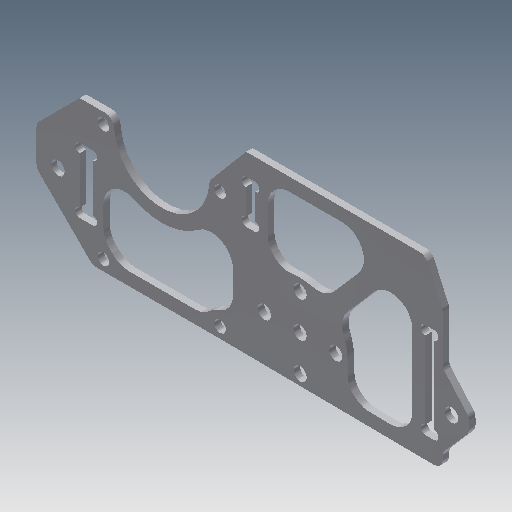
# Autodesk Inventor part: 付け根_メインフレーム_1_1
Saved by Autodesk Inventor 2017.3 (Build 213256000, 256)
## iProperties
Created: 2016-04-30
Part Number: 付け根_メインフレーム_1_1
Material: アルミニウム 2014-T4
Document SubType Name: Modeling
Designer: hiroaki
Density: 2.8 g/cm^3
Appearance: サテン
Mass: 7.66121 g
Surface Area: 47.3307 cm^2
Volume: 2.73615 cm^3
d0: 1.000 ul
d1: 3.000 mm
d2: 15.000 mm
d3: 5.000 mm
d4: 0.025 mm
d5: 2.100 mm
d6: 3.100 mm
d8: 15.000 mm
d9: 11.000 mm
d10: 2.000 mm
d11: 10.000 mm
d12: 5.000 mm
d13: 6.100 mm
d14: 1.000 mm
d15: 0.025 mm
d16: 2.100 mm
d17: 22.000 mm
d18: 5.000 mm
d19: 5.000 mm
d20: 15.000 mm
d21: 1.000 mm
d22: 27.000 mm
d23: 4.000 mm
d24: 2.000 mm
d25: 8.500 mm
d26: 8.500 mm
d28: 0.025 mm
d29: 2.100 mm
d30: 3.100 mm
d31: 1.500 mm
d32: 0.00 deg
d33: 2.100 mm
d34: 6.000 ul
d36: 360.00 deg
d38: 5.600 mm
d39: 0.250 mm
d40: 0.00 deg
Author: hiroaki
Autodesk Inventor part; units mm, degrees
ref_plane "YZ Plane" through (0, 0, 0) normal (1, 0, 0) x (0, 1, 0)
ref_plane "XZ Plane" through (0, 0, 0) normal (0, 1, 0) x (-1, 0, 0)
ref_plane "XY Plane" through (0, 0, 0) normal (0, 0, 1) x (1, 0, 0)
derived "下半身全体像_1_1.ipt"
sketch "スケッチ1" plane through (0, 0, 0) normal (0, 0, 1) x (1, 0, 0)
  circle A0 centre (0, 0) radius 10.5 construction
  line L0 (0, 0) -> (-12, 0) construction
  arc A1 (0, 16) -> (-12, 10.583) centre (0, 0) ccw construction
  arc A2 (-12, -10.583) -> (0, -16) centre (0, 0) ccw construction
  line L1 (0, 16) -> (39.5, 16) construction
  line L2 (39.5, 16) -> (39.5, -16) construction
  line L3 (39.5, -16) -> (0, -16) construction
  circle A3 centre (1, 13.5) radius 1.35 projected
  circle A4 centre (1, -13.5) radius 1.35 projected
  circle A5 centre (28, 13.5) radius 1.35 projected
  circle A6 centre (28, -13.5) radius 1.35 projected
  line L4 (1, 13.5) -> (1, -13.5) construction
  line L5 (1, -13.5) -> (28, -13.5) construction
  line L6 (1, 13.5) -> (28, 13.5) construction
  line L7 (28, 13.5) -> (28, -13.5) construction
  line L8 (0, 0) -> (1, 0) construction
  line L9 (32, 120) -> (32, 20) construction
  line L10 (0, 0) -> (0, 0) construction
  circle A7 centre (32, 120) radius 4.05 construction
  line L11 (0, 140) -> (0, 40) construction
  circle A8 centre (0, 40) radius 4.05 projected
  line L12 (0, 0) -> (0, -100) construction
  line L13 (32, 20) -> (32, -80) construction
  line L14 (0, 0) -> (0, 40) construction
  circle A9 centre (32, 20) radius 6.5 construction
  line L15 (32, 23.5218) -> (35.05, 21.7609) construction
  line L16 (35.05, 21.7609) -> (35.05, 18.2391) construction
  line L17 (35.05, 18.2391) -> (32, 16.4782) construction
  line L18 (32, 16.4782) -> (28.95, 18.2391) construction
  line L19 (28.95, 18.2391) -> (28.95, 21.7609) construction
  line L20 (28.95, 21.7609) -> (32, 23.5218) construction
  line L21 (21.5, 152) -> (61, 152) construction
  line L22 (61, 152) -> (61, 100.5) construction
  line L23 (61, 100.5) -> (21.5, 100.5) construction
  line L24 (21.5, 100.5) -> (21.5, 152) construction
  line L25 (21.5, 140) -> (61, 140) construction
  line L26 (16, 150.5) -> (66.5, 150.5) construction
  line L27 (66.5, 150.5) -> (66.5, 129.5) construction
  line L28 (66.5, 129.5) -> (16, 129.5) construction
  line L29 (16, 129.5) -> (16, 150.5) construction
  circle A10 centre (0, 140) radius 10.5 construction
  line L30 (-13.5, 139) -> (13.5, 139) construction
  line L31 (13.5, 139) -> (13.5, 112) construction
  line L32 (13.5, 112) -> (-13.5, 112) construction
  line L33 (-13.5, 112) -> (-13.5, 139) construction
  circle A11 centre (-13.5, 139) radius 1.35 projected
  circle A12 centre (13.5, 139) radius 1.35 projected
  circle A13 centre (-13.5, 112) radius 1.35 projected
  circle A14 centre (13.5, 112) radius 1.35 projected
  line L34 (-12, 10.583) -> (-12, -10.583) construction
  circle A15 centre (0, -100) radius 4.05 projected
  circle A16 centre (32, -80) radius 4.05 projected
  circle A17 centre (0, -100) radius 10.5 construction
  line L35 (32, -80) -> (0, -100) construction
  line L36 (45, -60.5) -> (77.5, -60.5) construction
  line L37 (77.5, -60.5) -> (77.5, -112) construction
  line L38 (77.5, -112) -> (45, -112) construction
  line L39 (45, -112) -> (45, -60.5) construction
  line L40 (45, -100) -> (77.5, -100) construction
  line L41 (39.5, -89.5) -> (83, -89.5) construction
  line L42 (83, -89.5) -> (83, -110.5) construction
  line L43 (83, -110.5) -> (39.5, -110.5) construction
  line L44 (39.5, -110.5) -> (39.5, -89.5) construction
  line L45 (1, -86.5) -> (28, -86.5) construction
  line L46 (28, -86.5) -> (28, -113.5) construction
  line L47 (28, -113.5) -> (1, -113.5) construction
  line L48 (1, -113.5) -> (1, -86.5) construction
  circle A18 centre (1, -86.5) radius 1.35 projected
  circle A19 centre (1, -113.5) radius 1.35 projected
  circle A20 centre (28, -113.5) radius 1.35 projected
  circle A21 centre (28, -86.5) radius 1.35 projected
  circle A22 centre (32, 20) radius 4.05 projected
  circle A23 centre (32, 20) radius 4.05 projected
  line L49 (10.583, 152) -> (-10.583, 152) construction
  line L50 (16, 140) -> (16, 100.5) construction
  line L51 (16, 100.5) -> (-16, 100.5) construction
  line L52 (-16, 100.5) -> (-16, 140) construction
  arc A24 (16, 140) -> (10.583, 152) centre (0, 140) ccw construction
  arc A25 (-10.583, 152) -> (-16, 140) centre (0, 140) ccw construction
  line L53 (-12, -89.417) -> (-12, -110.583) construction
  line L54 (0, -84) -> (39.5, -84) construction
  line L55 (39.5, -84) -> (39.5, -116) construction
  line L56 (39.5, -116) -> (0, -116) construction
  arc A26 (0, -84) -> (-12, -89.417) centre (0, -100) ccw construction
  arc A27 (-12, -110.583) -> (0, -116) centre (0, -100) ccw construction
  circle A28 centre (-8.5, 0) radius 1.35 projected
  circle A29 centre (0, 0) radius 8.5 construction
  line L57 (35.05, 121.7609) -> (35.05, 118.2391) construction
  line L58 (35.05, 118.2391) -> (32, 116.4782) construction
  line L59 (32, 116.4782) -> (28.95, 118.2391) construction
  line L60 (28.95, 118.2391) -> (28.95, 121.7609) construction
  line L61 (28.95, 121.7609) -> (32, 123.5218) construction
  line L62 (32, 123.5218) -> (35.05, 121.7609) construction
  line L63 (0, 152) -> (0, 140) construction
  line L64 (0, 140) -> (0, 139) construction
  line L65 (-19, 132.5) -> (-16, 132.5) construction
  line L66 (-16, 132.5) -> (-16, 117.5) construction
  line L67 (-16, 117.5) -> (-19, 117.5) construction
  line L68 (-19, 117.5) -> (-19, 132.5) construction
  line L69 (-19, 137.5) -> (-16, 137.5) construction
  line L70 (-16, 137.5) -> (-16, 112.5) construction
  line L71 (-16, 112.5) -> (-19, 112.5) construction
  line L72 (-19, 112.5) -> (-19, 137.5) construction
  line L73 (-15.975, 132.525) -> (-19.025, 132.525) construction
  line L74 (-19.025, 132.525) -> (-19.025, 117.475) construction
  line L75 (-19.025, 117.475) -> (-15.975, 117.475) construction
  line L76 (-15.975, 117.475) -> (-15.975, 132.525) construction
  circle A30 centre (-19.025, 131.475) radius 1.05 construction
  arc A31 (-19.025, 132.525) -> (-19.025, 130.425) centre (-19.025, 131.475) ccw
  line L77 (-19.025, 132.525) -> (-15.975, 132.525)
  arc A32 (-15.975, 130.425) -> (-15.975, 132.525) centre (-15.975, 131.475) ccw
  line L78 (-17.5, 132.525) -> (-17.5, 117.475) construction
  line L79 (-19, 125) -> (-16, 125) construction
  line L80 (-19.025, 130.425) -> (-19.025, 119.575)
  line L81 (-15.975, 130.425) -> (-15.975, 119.575)
  arc A33 (-19.025, 119.575) -> (-19.025, 117.475) centre (-19.025, 118.525) ccw
  arc A34 (-15.975, 117.475) -> (-15.975, 119.575) centre (-15.975, 118.525) ccw
  line L82 (-15.975, 117.475) -> (-19.025, 117.475)
  circle A35 centre (32, 120) radius 1.55
  circle A36 centre (-13.5, 139) radius 2.5 construction
  arc A37 (-10.8799, 138.3793) -> (10.8799, 138.3793) centre (0, 140) ccw
  line L83 (61, 136) -> (63, 136) construction
  line L84 (63, 136) -> (63, 114) construction
  line L85 (63, 114) -> (61, 114) construction
  line L86 (61, 114) -> (61, 136) construction
  line L87 (19.5, 145) -> (21.5, 145) construction
  line L88 (21.5, 145) -> (21.5, 135) construction
  line L89 (21.5, 135) -> (19.5, 135) construction
  line L90 (19.5, 135) -> (19.5, 145) construction
  line L91 (19.5, 150) -> (21.5, 150) construction
  line L92 (21.5, 150) -> (21.5, 130) construction
  line L93 (21.5, 130) -> (19.5, 130) construction
  line L94 (19.5, 130) -> (19.5, 150) construction
  line L95 (10.8799, 138.3793) -> (11.1317, 140.0691)
  circle A38 centre (13.5, 139) radius 2.5 construction
  line L96 (19.5, 150) -> (61, 150)
  line L97 (67.05, 124.5218) -> (70.1, 122.7609) construction
  line L98 (70.1, 122.7609) -> (70.1, 119.2391) construction
  line L99 (70.1, 119.2391) -> (67.05, 117.4782) construction
  line L100 (67.05, 117.4782) -> (64, 119.2391) construction
  line L101 (64, 119.2391) -> (64, 122.7609) construction
  line L102 (64, 122.7609) -> (67.05, 124.5218) construction
  line L103 (21.525, 145.025) -> (19.475, 145.025) construction
  line L104 (19.475, 145.025) -> (19.475, 134.975) construction
  line L105 (19.475, 134.975) -> (21.525, 134.975) construction
  line L106 (21.525, 134.975) -> (21.525, 145.025) construction
  circle A39 centre (19.475, 143.975) radius 1.05 construction
  arc A40 (19.475, 145.025) -> (19.475, 142.925) centre (19.475, 143.975) ccw
  line L107 (20.5, 134.975) -> (20.5, 145.025) construction
  line L108 (19.5, 140) -> (21.5, 140) construction
  line L109 (19.475, 145.025) -> (21.525, 145.025)
  arc A41 (21.525, 142.925) -> (21.525, 145.025) centre (21.525, 143.975) ccw
  line L110 (21.525, 142.925) -> (21.525, 137.075)
  line L111 (19.475, 142.925) -> (19.475, 137.075)
  arc A42 (19.475, 137.075) -> (19.475, 134.975) centre (19.475, 136.025) ccw
  line L112 (19.475, 134.975) -> (21.525, 134.975)
  arc A43 (21.525, 134.975) -> (21.525, 137.075) centre (21.525, 136.025) ccw
  line L113 (61, 150) -> (65, 141)
  line L114 (65, 141) -> (65, 129.5)
  line L115 (65, 141) -> (61, 141) construction
  line L116 (65, 129.5) -> (71.1, 122.5204)
  line L117 (71.1, 122.5204) -> (71.1, 119.4796)
  line L118 (71.1, 119.4796) -> (65, 112.5)
  circle A44 centre (67.05, 121) radius 4.05 construction
  line L119 (61, 109) -> (64.2641, 109) construction
  line L120 (63, 125) -> (61, 125) construction
  line L121 (21.5, 139) -> (61, 139) construction
  line L122 (61, 139) -> (61, 112) construction
  line L123 (61, 112) -> (21.5, 112) construction
  line L124 (21.5, 112) -> (21.5, 139) construction
  line L125 (65, 112.5) -> (65, 109)
  line L126 (61, 109) -> (13.4868, 109.5)
  line L127 (-29, 122.5) -> (-16, 109.5)
  line L128 (-16, 109.5) -> (13.4868, 109.5)
  circle A45 centre (-13.5, 112) radius 2.5 construction
  circle A46 centre (13.5, 112) radius 2.5 construction
  line L129 (63.025, 136.025) -> (60.975, 136.025) construction
  line L130 (60.975, 136.025) -> (60.975, 113.975) construction
  line L131 (60.975, 113.975) -> (63.025, 113.975) construction
  line L132 (63.025, 113.975) -> (63.025, 136.025) construction
  circle A47 centre (60.975, 134.975) radius 1.05 construction
  line L133 (62, 136.025) -> (62, 125) construction
  arc A48 (60.975, 136.025) -> (60.975, 133.925) centre (60.975, 134.975) ccw
  line L134 (60.975, 136.025) -> (63.025, 136.025)
  arc A49 (63.025, 133.925) -> (63.025, 136.025) centre (63.025, 134.975) ccw
  line L135 (60.975, 133.925) -> (60.975, 116.075)
  line L136 (63.025, 133.925) -> (63.025, 116.075)
  arc A50 (60.975, 116.075) -> (60.975, 113.975) centre (60.975, 115.025) ccw
  line L137 (60.975, 113.975) -> (63.025, 113.975)
  arc A51 (63.025, 113.975) -> (63.025, 116.075) centre (63.025, 115.025) ccw
  circle A52 centre (67.05, 121) radius 1.55
  line L138 (65, 109) -> (61, 109)
  line L139 (-11.3448, 141.5) -> (-10.8799, 138.3793)
  line L140 (-29, 131.5) -> (-19, 141.5)
  line L141 (-19, 141.5) -> (-11.3448, 141.5)
  circle A53 centre (32, 128.25) radius 1.55
  circle A54 centre (23.75, 120) radius 1.55
  circle A55 centre (32, 111.75) radius 1.55
  circle A56 centre (40.25, 120) radius 1.55
  circle A57 centre (32, 128.25) radius 2.75 construction
  circle A58 centre (32, 120) radius 5.5 construction
  line L142 (19.5, 150) -> (11.1317, 140.0691)
  circle A59 centre (19.5, 145) radius 1.5 construction
  line L143 (-21, 126.7321) -> (-21, 123.2679)
  line L144 (-21, 123.2679) -> (-24, 121.5359)
  line L145 (-24, 121.5359) -> (-27, 123.2679)
  line L146 (-27, 123.2679) -> (-27, 126.7321)
  line L147 (-27, 126.7321) -> (-24, 128.4641)
  line L148 (-24, 128.4641) -> (-21, 126.7321)
  circle A60 centre (-24, 125) radius 1.55
  line L149 (-29, 131.5) -> (-29, 122.5)
  point P0 (66.5, 140)
  point P1 (39.5, 0)
  point P2 (83, -100)
  point P3 (1, -100)
  point P4 (-12, -100)
  point P5 (39.5, -100)
  point P6 (71.1, 121)
  point P7 (-19.025, 125)
  dimension "d5" = 2.1
  dimension "d16" = 2.1
  dimension "d29" = 2.1
  dimension "d1" = 3
  dimension "d2" = 15
  dimension "d3" = 5
  dimension "d4" = 0.025
  dimension "d6" = 3.1
  dimension "d8" = 15
  dimension "d9" = 11
  dimension "d10" = 2
  dimension "d11" = 10
  dimension "d12" = 5
  dimension "d13" = 6.1
  dimension "d14" = 1
  dimension "d15" = 0.025
  dimension "d17" = 22
  dimension "d18" = 5
  dimension "d19" = 5
  dimension "d20" = 15
  dimension "d21" = 1
  dimension "d22" = 27
  dimension "d23" = 4
  dimension "d24" = 2
  dimension "d25" = 8.5
  dimension "d26" = 8.5
  dimension "d28" = 0.025
  dimension "d30" = 3.1
  dimension "d41" = 3.1
  dimension "d45" = 360
  dimension "d47" = 5.5
  dimension "d48" = 11
  dimension "d64" = 3
  dimension "d65" = 2
  dimension "d66" = 6
  dimension "d67" = 3.1
  dimension "d68" = 2
  dimension "d69" = 135
  constraints: 170 end point, 28 centre point, 26 point on circle, 20 parallel, 20 tangent, 19 horizontal, 18 collinear, 15 coincident, 15 midpoint, 11 symmetric about line, 11 vertical, 10 perpendicular, 10 point on line, 7 equal radius, 6 vertical alignment, 5 horizontal alignment, 55 other
  measures "d1" distance of L65.start L65.end
  measures "d2" distance of L67.end L65.start
  measures "d3" distance between parallel lines of L69 L65
  measures "d4" distance between parallel lines of L73 L65
  measures "d6" diameter of A35
  measures "d8" distance from line of A24.centre L79
  measures "d9" radius of A37
  measures "d10" distance of L83.start L83.end
  measures "d11" distance of L89.end L87.start
  measures "d12" distance between parallel lines of L91 L87
  measures "d13" distance between parallel lines of L101 L98
  measures "d14" distance between parallel lines of L101 L84
  measures "d15" distance between parallel lines of L103 L87
  measures "d17" distance of L83.end L84.end
  measures "d18" distance between parallel lines of L115 L83
  measures "d19" distance between parallel lines of L85 L119
  measures "d20" distance between parallel lines of L120 L25
  measures "d21" distance between parallel lines of L25 L121
  measures "d22" distance of L123.end L121.start
  measures "d23" distance from line of A44.centre L120
  measures "d24" distance between parallel lines of L114 L84
  measures "d25" vertical distance of L114.end point (67.05, 121)
  measures "d26" vertical distance of point (67.05, 121) L118.end
  measures "d28" distance between parallel lines of L129 L83
  measures "d30" diameter of A52
  measures "d41" diameter of A53
  measures "d47" diameter of A57
  measures "d48" diameter of A58
  measures "d64" diameter of A59
  measures "d65" distance between parallel lines of L68 L143
  measures "d66" distance between parallel lines of L146 L143
  measures "d67" diameter of A60
  measures "d68" distance between parallel lines of L149 L146
  measures "d69" angle of L141 L140
extrude "押し出し1" add sketch "スケッチ1" along normal blind 1.5 contours A37 L95 L142 L96 L113 L114 L116 L117 L118 L125 L138 L126 L128 L127 L149 L140 L141 L139 | L143 L144 L145 L146 L147 L148
sketch "スケッチ3" plane through (61, 150, 0) normal (0, 0, -1) x (-1, 0, 0)
  circle A0 centre (-6.05, -29) radius 1.55 projected
  line L0 (-8.85, -27.3834) -> (-6.05, -25.7668)
  line L1 (-6.05, -25.7668) -> (-3.25, -27.3834)
  line L2 (-3.25, -27.3834) -> (-3.25, -30.6166)
  line L3 (-3.25, -30.6166) -> (-6.05, -32.2332)
  line L4 (-6.05, -32.2332) -> (-8.85, -30.6166)
  line L5 (-8.85, -30.6166) -> (-8.85, -27.3834)
  circle A1 centre (-6.05, -26.8168) radius 1.05
  circle A2 centre (-7.9407, -27.9084) radius 1.05
  circle A3 centre (-7.9407, -30.0916) radius 1.05
  circle A4 centre (-6.05, -31.1832) radius 1.05
  circle A5 centre (-4.1593, -30.0916) radius 1.05
  circle A6 centre (-4.1593, -27.9084) radius 1.05
  circle A7 centre (85, -25) radius 1.55 projected
  line L6 (87.8, -23.3834) -> (87.8, -26.6166)
  line L7 (87.8, -26.6166) -> (85, -28.2332)
  line L8 (85, -28.2332) -> (82.2, -26.6166)
  line L9 (82.2, -26.6166) -> (82.2, -23.3834)
  line L10 (82.2, -23.3834) -> (85, -21.7668)
  line L11 (85, -21.7668) -> (87.8, -23.3834)
  circle A8 centre (85, -22.8168) radius 1.05
  circle A9 centre (83.1093, -23.9084) radius 1.05
  circle A10 centre (83.1093, -26.0916) radius 1.05
  circle A11 centre (85, -27.1832) radius 1.05
  circle A12 centre (86.8907, -26.0916) radius 1.05
  circle A13 centre (86.8907, -23.9084) radius 1.05
  point P0 (61, -150)
  point P1 (-6.05, -29)
  point P2 (-8.85, -27.3834)
  point P3 (-8.85, -30.6166)
  point P4 (-3.25, -30.6166)
  point P5 (-3.25, -27.3834)
  point P6 (85, -25)
  point P7 (82.2, -23.3834)
  point P8 (82.2, -26.6166)
  point P9 (85, -28.2332)
  point P10 (87.8, -26.6166)
  point P11 (87.8, -23.3834)
  dimension "d33" = 2.1
  dimension "d74" = 2.1
  dimension "d36" = 360
  dimension "d38" = 5.6
  dimension "d77" = 360
  constraints: 24 end point, 6 vertical alignment, 2 coincident, 2 vertical, 1 equal length, 96 other
  measures "d38" distance between parallel lines of L2 L5
extrude "押し出し2" cut sketch "スケッチ3" against normal blind 0.25 contours A0 A6 L2 A5 | A6 A0 | A0 A6 L1 L2 | A5 L2 L3 A0 | A0 A5 | A0 A1 L1 A6 | L2 A6 | A5 L3 A4 A0 | A5 L2 | A1 A0 | A0 A1 L0 L1 | A6 L1 | A4 L3 L4 A0 | A0 A4 | L3 A5 | A0 A2 L0 A1 | L1 A1 | A4 L4 A3 A0 | A4 L3 | A2 A0 | A0 A2 L5 L0 | A1 L0 | A3 L4 L5 A0 | A0 A3 | L4 A4 | A0 A3 L5 A2 | L0 A2 | A3 L4 | A2 L5 | L5 A3 | A7 A13 L6 A12 | A13 A7 | A7 A13 L11 L6 | A12 L6 L7 A7 | A7 A12 | A7 A8 L11 A13 | L6 A13 | A12 L7 A11 A7 | A12 L6 | A8 A7 | A7 A8 L10 L11 | A13 L11 | A11 L7 L8 A7 | A7 A11 | L7 A12 | A7 A9 L10 A8 | L11 A8 | A11 L8 A10 A7 | A11 L7 | A9 A7 | A7 A9 L9 L10 | A8 L10 | A10 L8 L9 A7 | A7 A10 | L8 A11 | A7 A10 L9 A9 | L10 A9 | A10 L8 | A9 L9 | L9 A10
sketch "スケッチ4" plane through (12.611, 150, 1.5) normal (0, 0, 1) x (1, 0, 0)
  line L0 (-28.586, -32.525) -> (-31.636, -32.525) projected
  line L1 (48.364, -13.975) -> (50.414, -13.975) projected
  line L2 (50.414, -36.025) -> (48.364, -36.025) projected
  line L3 (6.864, -4.975) -> (8.914, -4.975) projected
  line L4 (8.914, -15.025) -> (6.864, -15.025) projected
  circle A0 centre (19.389, -30) radius 1.55 projected
  circle A1 centre (0.889, -38) radius 1.35 projected
  circle A2 centre (-26.111, -38) radius 1.35 projected
  circle A3 centre (0.889, -11) radius 1.35 projected
  line L5 (-41.611, -18.5) -> (-41.611, -27.5)
  line L6 (-28.611, -40.5) -> (0.8758, -40.5) projected
  line L7 (0.8758, -40.5) -> (48.389, -41) projected
  line L8 (48.389, 0) -> (6.889, 0) projected
  arc A4 (-23.491, -11.6207) -> (-1.7311, -11.6207) centre (-12.611, -10) ccw projected
  line L9 (-26.111, -13.7081) -> (-26.111, -35)
  arc A5 (-23.153, -37.5) -> (-26.111, -35) centre (-26.111, -38) ccw
  line L10 (-28.586, -17.475) -> (-31.636, -17.475) construction
  line L11 (-30.111, -17.475) -> (-30.111, -32.525) construction
  arc A6 (-26.111, -13.7081) -> (0.8054, -14) centre (-12.611, -10) ccw
  line L12 (0.8054, -14) -> (3.889, -14)
  line L13 (3.889, -14) -> (3.889, -35)
  line L14 (-23.153, -37.5) -> (-2.0691, -37.5)
  line L15 (3.889, -35) -> (0.889, -35)
  arc A7 (0.889, -35) -> (-2.0691, -37.5) centre (0.889, -38) ccw
  line L16 (7.889, -4.975) -> (7.889, -15.025) construction
  line L17 (11.889, -3) -> (11.889, -21.9533)
  line L18 (11.889, -3) -> (40.1001, -3)
  arc A8 (24.9528, -20.5109) -> (11.889, -21.9533) centre (19.389, -30) ccw
  line L19 (49.389, -13.975) -> (49.389, -36.025) construction
  line L20 (45.389, -37.9683) -> (30.389, -37.8104)
  line L21 (40.1001, -3) -> (24.9528, -20.5109)
  line L22 (30.389, -37.8104) -> (30.389, -30)
  arc A9 (30.389, -30) -> (27.978, -23.1278) centre (19.389, -30) ccw
  line L23 (27.978, -23.1278) -> (45.389, -3)
  line L24 (45.389, -3) -> (45.389, -37.9683)
  line L25 (19.389, -30) -> (42.7445, -3) construction
  line L26 (40.1001, -3) -> (45.389, -3) construction
  circle A10 centre (19.389, -21.75) radius 1.55 projected
  circle A11 centre (19.389, -21.75) radius 2.75 construction
  point P0 (0, 0)
  point P1 (-12.611, -150)
  dimension "d49" = 3
  dimension "d50" = 4
  dimension "d51" = 3
  dimension "d52" = 3
  dimension "d53" = 4
  dimension "d54" = 3
  dimension "d56" = 4
  dimension "d57" = 3
  dimension "d59" = 3
  dimension "d72" = 4
  dimension "d73" = 4
  dimension "d79" = 5.5
  constraints: 36 end point, 10 point on circle, 7 midpoint, 6 centre point, 6 coincident, 4 horizontal, 3 parallel, 3 tangent, 3 vertical, 2 equal radius, 1 horizontal alignment, 1 perpendicular, 1 other
  measures "d49" radius of A5
  measures "d50" distance between parallel lines of L11 L9
  measures "d51" radial gap between concentric circles of A6 A4
  measures "d52" distance from line of A3.centre L12
  measures "d53" distance between parallel lines of L13 L16
  measures "d54" distance between parallel lines of L14 L6
  measures "d56" distance between parallel lines of L17 L16
  measures "d57" distance between parallel lines of L8 L18
  measures "d59" distance between parallel lines of L7 L20
  measures "d72" distance between parallel lines of L19 L24
  measures "d73" distance between parallel lines of L23 L21
  measures "d79" diameter of A11
extrude "押し出し3" cut sketch "スケッチ4" against normal blind 10 contours A6 L12 L13 L15 A7 L14 A5 L9 | L18 L21 A8 L17 | L20 L22 A9 L23 L24
fillet "フィレット1" radius 5 15 edges at (-13.5, 136.2919, 0.75) (13.4164, 136, 0.75) (16.5, 136, 0.75) (16.5, 115, 0.75) (10.542, 112.5, 0.75) (-13.5, 115, 0.75) (-10.542, 112.5, 0.75) (24.5, 128.0467, 0.75) (24.5, 147, 0.75) (52.7111, 147, 0.75) (58, 112.0317, 0.75) (43, 112.1896, 0.75) (37.5639, 129.4891, 0.75) (40.5891, 126.8722, 0.75) (58, 147, 0.75)
fillet "フィレット2" radius 2 11 edges at (-11.3448, 141.5, 0.75) (61, 150, 0.75) (65, 129.5, 0.75) (65, 141, 0.75) (71.1, 122.5204, 0.75) (71.1, 119.4796, 0.75) (65, 112.5, 0.75) (65, 109, 0.75) (-29, 122.5, 0.75) (-16, 109.5, 0.75) (-29, 131.5, 0.75)
equation "\"d19\" = d18"
equation "\"d26\" = d25"
